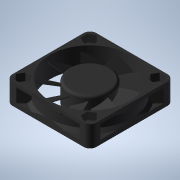
# Autodesk Inventor part: ZHJ06-4010M2
Saved by Autodesk Inventor 2021 (Build 250183000, 183)
## iProperties
Created: 2025-10-10
Part Number: ZHJ06-4010M2
Material: Generic
Catalog Web Link: www.cadenas.de
Description: ZHJ06-Fan · Economic · DC Axial Fan
Vendor: YIHEDA
Document SubType Name: Modeling
Designer: psAdmin
Manufacturer: YIHEDA
Mass: 5.33823 g
Surface Area: 85.8793 cm^2
Volume: 5.33823 cm^3
Density: 1 g/cm^3
Appearance: PSOLRGB-175-175-175
Category: PARTsolutions
Company: YIHEDA
Title: ZHJ06-4010M2
Author: Cadenas PARTsolutions
Comments: Fan · Economic · DC Axial Fan
PSOL_IDENT_0: {$CADENAS_DATA/23d-libs/yiheda/yhd_electric/fx01/fx01.40/fx01.40.01/zhj06.prj},165 {VTYP=3D},{NB=ZHJ
PSOL_IDENT_1: 06-4010M2},{LINA=ZHJ06-4010M2},{NN=ZHJ06},{DATE=31.08.2025 11:19:24},{GEOMDATE=07.08.2025 07:53:25},
PSOL_IDENT_2: {VERSION=},{LINEID=10},{WBVAR=ED},{WBNUMERIC=}  {NB=ZHJ06-4010M2},{LINA=ZHJ06-4010M2},{KT=DUMMY},{CO
PSOL_IDENT_3: DE=ZHJ06},{TYPE=Axial flow fan · DC type},{MAT=PBT},{BEA=Double ball bearing},{FRG=UL94V-0},{ED=4010
PSOL_IDENT_4: M2},{LWH=40×40×10},{ADA=Protective net ZHJ42  filterZHJ41 or louverZHJ43},{SLT=M(standard)},{INV=DC2
PSOL_IDENT_5: 4V},{ELE=0.06},{RS=6000},{AIR=8.00},{WP=4.50},{NOI=28.00},{WEI=20},{NENN=ZHJ06-4010M2},{CNSTYPECODE=
PSOL_IDENT_6: ZHJ06-4010M2},{WEB=https://brand.yhdfa.com/products/ZHJ06?productModel=ZHJ06-4010M2},{LINK=website l
PSOL_IDENT_7: ink}
NB: ZHJ06-4010M2
NN: ZHJ06
NT: Fan · Economic · DC Axial Fan
NBSYN: $NENN.
LINA: ZHJ06-4010M2
CATALOG: YIHEDA
ROWDESC: ZHJ06-4010M2
CODE: ZHJ06
TYPE: Axial flow fan · DC type
MAT: PBT
BEA: Double ball bearing
FRG: UL94V-0
ED: 4010M2
LWH: 40×40×10
ADA: Protective net ZHJ42  filterZHJ41 or louverZHJ43
SLT: M(standard)
INV: DC24V
ELE: 0.06
RS: 6000
AIR: 8
WP: 4.5
NOI: 28
WEI: 20
LINK: website link
SUPPLIER: YIHEDA
ARTICLENO: ZHJ06-4010M2
BOMINFO: ZHJ06-4010M2
CREATOR: CADENAS GmbH
Autodesk Inventor part; units mm, degrees
ref_plane "YZ Plane" through (0, 0, 0) normal (1, 0, 0) x (0, 1, 0)
ref_plane "XZ Plane" through (0, 0, 0) normal (0, 1, 0) x (-1, 0, 0)
ref_plane "XY Plane" through (0, 0, 0) normal (0, 0, 1) x (1, 0, 0)
sketch "__1" plane through (0, 0, 0) normal (0, 0, 1) x (1, 0, 0)
  line L0 (0, 0) -> (0, 9.6)
  line L1 (0, 9.6) -> (10, 9.6)
  line L2 (10, 9.6) -> (10, 2.6)
  line L3 (10, 2.6) -> (9.3, 2.6)
  line L4 (9.3, 2.6) -> (9.3, 8.1)
  arc A0 (9.3, 8.1) -> (8.8, 8.6) centre (8.8, 8.1) ccw
  line L5 (8.8, 8.6) -> (6.5, 8.6)
  arc A1 (6.5, 8.6) -> (6, 8.1) centre (6.5, 8.1) ccw
  line L6 (6, 8.1) -> (6, 6.6)
  line L7 (6, 6.6) -> (7.8, 6.6)
  line L8 (7.8, 6.6) -> (7.8, 4.6)
  line L9 (7.8, 4.6) -> (6, 4.6)
  line L10 (6, 4.6) -> (6, 1.2)
  line L11 (6, 1.2) -> (10, 1.2)
  line L12 (10, 1.2) -> (10, 0)
  line L13 (10, 0) -> (0, 0)
  line L14 (0, 0) -> (0, 9.6)
  constraints: 30 end point, 4 point on circle, 2 centre point
revolve "Revolution1" add sketch "__1" angle 360 about axis through (0, 0, 0) along (0, -1, 0)
sketch "__2" plane through (0, 0, 0) normal (0, 0, 1) x (1, 0, 0)
  line L0 (-4.75, 8.142) -> (-4.75, 7.8)
  line L1 (-4.75, 7.8) -> (4.75, 2.6)
  line L2 (4.75, 2.6) -> (4.75, 2.942)
  line L3 (4.75, 2.942) -> (-4.75, 8.142)
  constraints: 8 end point
extrude "Extrusion1" add sketch "__2" against normal blind 22.5
sketch "__3" plane through (0, 0, 0) normal (0.6427876, 0, 0.7660444) x (0.7660444, 0, -0.6427876)
  line L0 (-4.75, 8.142) -> (-4.75, 7.8)
  line L1 (-4.75, 7.8) -> (4.75, 2.6)
  line L2 (4.75, 2.6) -> (4.75, 2.942)
  line L3 (4.75, 2.942) -> (-4.75, 8.142)
  constraints: 8 end point
sketch "__4" plane through (0, 0, 0) normal (0.9848078, 0, 0.1736482) x (0.1736482, 0, -0.9848078)
  line L0 (-4.75, 8.142) -> (-4.75, 7.8)
  line L1 (-4.75, 7.8) -> (4.75, 2.6)
  line L2 (4.75, 2.6) -> (4.75, 2.942)
  line L3 (4.75, 2.942) -> (-4.75, 8.142)
  constraints: 8 end point
sketch "__5" plane through (0, 0, 0) normal (0.8660254, 0, -0.5) x (-0.5, 0, -0.8660254)
  line L0 (-4.75, 8.142) -> (-4.75, 7.8)
  line L1 (-4.75, 7.8) -> (4.75, 2.6)
  line L2 (4.75, 2.6) -> (4.75, 2.942)
  line L3 (4.75, 2.942) -> (-4.75, 8.142)
  constraints: 8 end point
sketch "__6" plane through (0, 0, 0) normal (0.3420201, 0, -0.9396926) x (-0.9396926, 0, -0.3420201)
  line L0 (-4.75, 8.142) -> (-4.75, 7.8)
  line L1 (-4.75, 7.8) -> (4.75, 2.6)
  line L2 (4.75, 2.6) -> (4.75, 2.942)
  line L3 (4.75, 2.942) -> (-4.75, 8.142)
  constraints: 8 end point
sketch "__7" plane through (0, 0, 0) normal (-0.3420201, 0, -0.9396926) x (-0.9396926, 0, 0.3420201)
  line L0 (-4.75, 8.142) -> (-4.75, 7.8)
  line L1 (-4.75, 7.8) -> (4.75, 2.6)
  line L2 (4.75, 2.6) -> (4.75, 2.942)
  line L3 (4.75, 2.942) -> (-4.75, 8.142)
  constraints: 8 end point
sketch "__8" plane through (0, 0, 0) normal (-0.8660254, 0, -0.5) x (-0.5, 0, 0.8660254)
  line L0 (-4.75, 8.142) -> (-4.75, 7.8)
  line L1 (-4.75, 7.8) -> (4.75, 2.6)
  line L2 (4.75, 2.6) -> (4.75, 2.942)
  line L3 (4.75, 2.942) -> (-4.75, 8.142)
  constraints: 8 end point
sketch "__9" plane through (0, 0, 0) normal (-0.9848078, 0, 0.1736482) x (0.1736482, 0, 0.9848078)
  line L0 (-4.75, 8.142) -> (-4.75, 7.8)
  line L1 (-4.75, 7.8) -> (4.75, 2.6)
  line L2 (4.75, 2.6) -> (4.75, 2.942)
  line L3 (4.75, 2.942) -> (-4.75, 8.142)
  constraints: 8 end point
sketch "__10" plane through (0, 0, 0) normal (-0.6427876, 0, 0.7660444) x (0.7660444, 0, 0.6427876)
  line L0 (-4.75, 8.142) -> (-4.75, 7.8)
  line L1 (-4.75, 7.8) -> (4.75, 2.6)
  line L2 (4.75, 2.6) -> (4.75, 2.942)
  line L3 (4.75, 2.942) -> (-4.75, 8.142)
  constraints: 8 end point
extrude "Extrusion2" add sketch "__3" against normal blind 22.5
extrude "Extrusion3" add sketch "__4" against normal blind 22.5
extrude "Extrusion4" add sketch "__5" against normal blind 22.5
extrude "Extrusion5" add sketch "__6" against normal blind 22.5
extrude "Extrusion6" add sketch "__7" against normal blind 22.5
extrude "Extrusion7" add sketch "__8" against normal blind 22.5
extrude "Extrusion8" add sketch "__9" against normal blind 22.5
extrude "Extrusion9" add sketch "__10" against normal blind 22.5
sketch "__11" plane through (0, 9.6, 0) normal (0, 1, 0) x (1, 0, 0)
  circle A0 centre (0, 0) radius 25
  circle A1 centre (0, 0) radius 18.5
  constraints: 2 centre point
extrude "Extrusion10" cut sketch "__11" against normal blind 12
sketch "__12" plane through (0, 0, 0) normal (0, 0, 1) x (1, 0, 0)
  line L0 (0, 0) -> (0, 9.6)
  line L1 (6, 4.6) -> (6, 2.6)
  line L2 (6, 2.6) -> (9.3, 2.6)
  line L3 (9.3, 2.6) -> (9.3, 8.1)
  arc A0 (9.3, 8.1) -> (8.8, 8.6) centre (8.8, 8.1) ccw
  line L4 (8.8, 8.6) -> (6.5, 8.6)
  arc A1 (6.5, 8.6) -> (6, 8.1) centre (6.5, 8.1) ccw
  line L5 (6, 8.1) -> (6, 6.6)
  line L6 (6, 6.6) -> (7.8, 6.6)
  line L7 (7.8, 6.6) -> (7.8, 4.6)
  line L8 (7.8, 4.6) -> (6, 4.6)
  constraints: 18 end point, 4 point on circle, 2 centre point
revolve "Revolution2" cut sketch "__12" angle 360 about axis through (0, 0, 0) along (0, -1, 0)
sketch "__13" plane through (0, 9.6, 0) normal (0, 1, 0) x (1, 0, 0)
  line L0 (-18.433, -1.573) -> (-9.491, -3.1498)
  arc A0 (-9.491, -3.1498) -> (-6.1533, -7.8827) centre (0, 0) ccw
  arc A1 (-13.1094, -13.0535) -> (-6.1533, -7.8827) centre (-36.3526, 25.479) ccw
  line L1 (-13.1094, -13.0535) -> (-5.2459, -8.5135)
  arc A2 (-5.2459, -8.5135) -> (0.3532, -9.9938) centre (0, 0) ccw
  arc A3 (-1.6517, -18.4261) -> (0.3532, -9.9938) centre (-44.2252, -3.8489) ccw
  line L2 (-1.6517, -18.4261) -> (1.4538, -9.8938)
  arc A4 (1.4538, -9.8938) -> (6.6945, -7.4286) centre (0, 0) ccw
  arc A5 (10.5788, -15.1769) -> (6.6945, -7.4286) centre (-31.4045, -31.3759) ccw
  line L3 (10.5788, -15.1769) -> (7.4733, -6.6446)
  arc A6 (7.4733, -6.6446) -> (9.9033, -1.3875) centre (0, 0) ccw
  arc A7 (17.8594, -4.8263) -> (9.9033, -1.3875) centre (-3.8892, -44.2217) ccw
  line L4 (17.8594, -4.8263) -> (9.9959, -0.2863)
  arc A8 (9.9959, -0.2863) -> (8.4782, 5.3028) centre (0, 0) ccw
  arc A9 (16.7833, 7.7826) -> (8.4782, 5.3028) centre (25.4459, -36.3757) ccw
  line L5 (16.7833, 7.7826) -> (7.8413, 6.2059)
  arc A10 (7.8413, 6.2059) -> (3.0861, 9.5119) centre (0, 0) ccw
  arc A11 (7.8542, 16.75) -> (3.0861, 9.5119) centre (42.8746, -11.5091) ccw
  line L6 (7.8542, 16.75) -> (2.0177, 9.7943)
  arc A12 (2.0177, 9.7943) -> (-3.75, 9.2702) centre (0, 0) ccw
  arc A13 (-4.75, 17.8798) -> (-3.75, 9.2702) centre (40.2417, 18.7427) ccw
  line L7 (-4.75, 17.8798) -> (-4.75, 8.7999)
  arc A14 (-4.75, 8.7999) -> (-8.8315, 4.691) centre (0, 0) ccw
  arc A15 (-15.1316, 10.6435) -> (-8.8315, 4.691) centre (18.7793, 40.2247) ccw
  line L8 (-15.1316, 10.6435) -> (-9.2952, 3.6878)
  arc A16 (-9.2952, 3.6878) -> (-9.7806, -2.0833) centre (0, 0) ccw
  arc A17 (-18.433, -1.573) -> (-9.7806, -2.0833) centre (-11.4701, 42.885) ccw
  circle A18 centre (0, 0) radius 9.7
  constraints: 36 point on circle, 19 centre point, 18 end point
extrude "Extrusion11" cut sketch "__13" against normal blind 3
sketch "__14" plane through (0, 2.6, 0) normal (0, -1, 0) x (1, 0, 0)
  line L0 (-17.8594, 4.8263) -> (-9.9959, 0.2863)
  arc A0 (-9.9959, 0.2863) -> (-9.2049, -3.9078) centre (0, 0) ccw
  arc A1 (-16.7833, -7.7826) -> (-9.2049, -3.9078) centre (-21.8904, 11.5543) ccw
  line L1 (-16.7833, -7.7826) -> (-7.8413, -6.2059)
  arc A2 (-7.8413, -6.2059) -> (-4.5395, -8.9103) centre (0, 0) ccw
  arc A3 (-7.8542, -16.75) -> (-4.5395, -8.9103) centre (-24.196, -5.2198) ccw
  line L2 (-7.8542, -16.75) -> (-2.0177, -9.7943)
  arc A4 (-2.0177, -9.7943) -> (2.25, -9.7436) centre (0, 0) ccw
  arc A5 (4.75, -17.8798) -> (2.25, -9.7436) centre (-15.18, -19.5515) ccw
  line L3 (4.75, -17.8798) -> (4.75, -8.7999)
  arc A6 (4.75, -8.7999) -> (7.9867, -6.0177) centre (0, 0) ccw
  arc A7 (15.1316, -10.6435) -> (7.9867, -6.0177) centre (0.9389, -24.7348) ccw
  line L4 (15.1316, -10.6435) -> (9.2952, -3.6878)
  arc A8 (9.2952, -3.6878) -> (9.9863, 0.5239) centre (0, 0) ccw
  arc A9 (18.433, 1.573) -> (9.9863, 0.5239) centre (16.6185, -18.3445) ccw
  line L5 (18.433, 1.573) -> (9.491, 3.1498)
  arc A10 (9.491, 3.1498) -> (7.3132, 6.8204) centre (0, 0) ccw
  arc A11 (13.1094, 13.0535) -> (7.3132, 6.8204) centre (24.5221, -3.3705) ccw
  line L6 (13.1094, 13.0535) -> (5.2459, 8.5135)
  arc A12 (5.2459, 8.5135) -> (1.2182, 9.9255) centre (0, 0) ccw
  arc A13 (1.6517, 18.4261) -> (1.2182, 9.9255) centre (20.9515, 13.1805) ccw
  line L7 (1.6517, 18.4261) -> (-1.4538, 9.8938)
  arc A14 (-1.4538, 9.8938) -> (-5.4468, 8.3864) centre (0, 0) ccw
  arc A15 (-10.5788, 15.1769) -> (-5.4468, 8.3864) centre (7.5776, 23.5642) ccw
  line L8 (-10.5788, 15.1769) -> (-7.4733, 6.6446)
  arc A16 (-7.4733, 6.6446) -> (-9.5632, 2.9232) centre (0, 0) ccw
  arc A17 (-17.8594, 4.8263) -> (-9.5632, 2.9232) centre (-9.3421, 22.922) ccw
  circle A18 centre (0, 0) radius 9.7
  constraints: 36 point on circle, 19 centre point, 18 end point
extrude "Extrusion12" cut sketch "__14" against normal blind 2.5
sketch "__15" plane through (0, 0, 0) normal (0, 0, 1) x (1, 0, 0)
  line L0 (0, 0) -> (0, 9.6)
  line L1 (9.3, 2.6) -> (10, 2.6)
  line L2 (10, 2.6) -> (10, 9.6)
  line L3 (10, 9.6) -> (9.3, 9.6)
  line L4 (9.3, 9.6) -> (9.3, 2.6)
  constraints: 10 end point
revolve "Revolution3" add sketch "__15" angle 360 about axis through (0, 0, 0) along (0, -1, 0)
sketch "__16" plane through (0, 0, 0) normal (0, 0, 1) x (1, 0, 0)
  line L0 (0, 0) -> (0, 9.6)
  arc A0 (10, 8.4) -> (8.8, 9.6) centre (8.8, 8.4) ccw
  line L1 (10, 8.4) -> (10, 9.6)
  line L2 (10, 9.6) -> (8.8, 9.6)
  constraints: 6 end point, 2 point on circle, 1 centre point
revolve "Revolution4" cut sketch "__16" angle 360 about axis through (0, 0, 0) along (0, -1, 0)
sketch "__17" plane through (0, 0, 0) normal (0, -1, 0) x (1, 0, 0)
  arc A0 (1.36, 9.9071) -> (-11.2, 15.348) centre (-13.231, -6.5581) ccw
  line L0 (1.36, 9.9071) -> (8.6603, 5)
  arc A1 (8.6603, 5) -> (-7.86, 17.298) centre (-13.8557, -8.0013) ccw
  arc A2 (-7.86, 17.298) -> (-11.2, 15.348) centre (0, 0) ccw
  constraints: 6 point on circle, 3 centre point, 2 end point
extrude "Extrusion13" add sketch "__17" against normal blind 1.1
pattern_circular "Circular Pattern1" count 3 over 360 about axis through (0, 0, 0) along (0, -1, 0) of "Extrusion13"
sketch "__19" plane through (0, 0, 0) normal (0, -1, 0) x (1, 0, 0)
  line L0 (-20, 17) -> (-20, -17)
  arc A0 (-20, -17) -> (-17, -20) centre (-17, -17) ccw
  line L1 (-17, -20) -> (17, -20)
  arc A1 (17, -20) -> (20, -17) centre (17, -17) ccw
  line L2 (20, -17) -> (20, 17)
  arc A2 (20, 17) -> (17, 20) centre (17, 17) ccw
  line L3 (17, 20) -> (-17, 20)
  arc A3 (-17, 20) -> (-20, 17) centre (-17, 17) ccw
  circle A4 centre (16, -16) radius 1.7
  circle A5 centre (16, 16) radius 1.7
  circle A6 centre (-16, -16) radius 1.7
  circle A7 centre (-16, 16) radius 1.7
  circle A8 centre (0, 0) radius 19
  constraints: 9 centre point, 8 end point, 8 point on circle
extrude "Extrusion14" add sketch "__19" against normal blind 10
sketch "__20" plane through (0, 0, 0) normal (0, 0, 1) x (1, 0, 0)
  line L0 (0, 2) -> (0, 8.48)
  line L1 (20, 7.4193) -> (20, 3.4142)
  line L2 (20, 3.4142) -> (21.4142, 2)
  line L3 (21.4142, 2) -> (30, 2)
  line L4 (30, 2) -> (30, 8.48)
  line L5 (30, 8.48) -> (21.0607, 8.48)
  line L6 (21.0607, 8.48) -> (20, 7.4193)
  constraints: 14 end point
revolve "Revolution5" cut sketch "__20" angle 360 about axis through (0, 2, 0) along (0, -1, 0)
sketch "__21" plane through (0, 2, 0) normal (0, 1, 0) x (1, 0, 0)
  arc A0 (16.3988, 11.449) -> (11.449, 16.3988) centre (0, 0) ccw
  line L0 (16.3988, 11.449) -> (20, 15.0503)
  line L1 (20, 15.0503) -> (20, 17)
  arc A1 (20, 17) -> (17, 20) centre (17, 17) ccw
  line L2 (17, 20) -> (15.0503, 20)
  line L3 (15.0503, 20) -> (11.449, 16.3988)
  circle A2 centre (16, 16) radius 1.7
  constraints: 8 end point, 4 point on circle, 3 centre point
extrude "Extrusion15" add sketch "__21" along normal blind 6.48
pattern_circular "Circular Pattern2" count 4 over 360 about axis through (0, 2, 0) along (0, 1, 0) of "Extrusion15"
sketch "__23" plane through (0, 10, 0) normal (0, 1, 0) x (-1, 0, 0)
  line L0 (-18.75, 14.4123) -> (-16, 12.8246)
  line L1 (-16, 12.8246) -> (-13.25, 14.4123)
  line L2 (-13.25, 14.4123) -> (-13.25, 17.5877)
  line L3 (-13.25, 17.5877) -> (-16, 19.1754)
  line L4 (-16, 19.1754) -> (-18.75, 17.5877)
  line L5 (-18.75, 17.5877) -> (-18.75, 14.4123)
  constraints: 12 end point
extrude "Extrusion16" cut sketch "__23" against normal blind 3.5
pattern_circular "Circular Pattern3" count 4 over 360 about axis through (0, 10, 0) along (0, 1, 0) of "Extrusion16"
body "Solid1"
